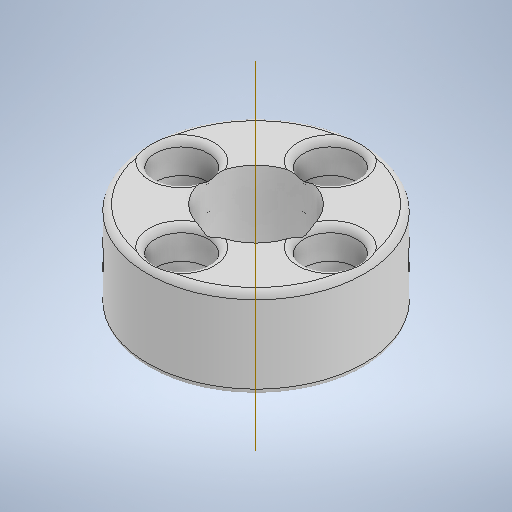
# Autodesk Inventor part: fixation_harbre_moteur_v2
Saved by Autodesk Inventor 2025.1 (Build 291241000, 241)
## iProperties
Created: 2025-05-14
Part Number: fixation_harbre_moteur_v2
Material: Générique
Document SubType Name: Modeling
Designer: chapuzet
Density: 1 g/cm^3
Appearance: Par défaut
Author: chapuzet
Autodesk Inventor part; units mm, degrees
ref_plane "XZ Plane" through (0, 0, 0) normal (0, 1, 0) x (-1, 0, 0)
sketch "Esquisse1" plane through (0, 0, 0) normal (0, 1, 0) x (-1, 0, 0)
  circle A0 centre (0, 0) radius 17.5
  circle A1 centre (0, 0) radius 12
  circle A2 centre (0, -12) radius 2
  circle A3 centre (12, 0) radius 2
  circle A4 centre (0, 12) radius 2
  circle A5 centre (-12, 0) radius 2
  dimension "d1" = 24
  dimension "d0" = 35
  dimension "d2" = 4
  dimension "d11" = 360
  constraints: 5 centre point, 2 coincident, 1 vertical alignment, 11 other
  measures "d0" diameter of A0
  measures "d2" diameter of A2
extrude "Extrusion1" add sketch "Esquisse1" along normal blind 14.5 contours A0 | A3 A1 A2 A5 A4
sketch "Esquisse2" plane through (0, 14.5, 0) normal (0, 1, 0) x (1, 0, 0)
  circle A0 centre (0, 12) radius 2 projected
  circle A1 centre (0, 12) radius 4.25
  circle A2 centre (-12, 0) radius 4.25
  circle A3 centre (0, -12) radius 4.25
  circle A4 centre (12, 0) radius 4.25
  point P0 (0, 0)
  dimension "d13" = 8.5
  dimension "d16" = 360
  constraints: 4 centre point, 1 coincident, 9 other
  measures "d13" diameter of A1
extrude "Extrusion2" cut sketch "Esquisse2" against normal blind 6
sketch "Esquisse3" plane through (0, 14.5, 0) normal (0, 1, 0) x (1, 0, 0)
  circle A0 centre (0, 0) radius 7.7
  dimension "d20" = 15.4
  constraints: 1 centre point, 1 coincident
  measures "d20" diameter of A0
extrude "Extrusion3" cut sketch "Esquisse3" against normal through all
fillet "Congé2" radius 1 14 edges at (17.5, 0, 0) (14, 0, 0) (2, 0, -12) (-10, 0, 0) (2, 0, 12) (17.5, 14.5, 0) (-16.25, 8.5, 0) (-16.25, 14.5, 0) (-4.25, 8.5, 12) (-4.25, 14.5, 12) (-4.25, 8.5, -12) (-4.25, 14.5, -12) (7.75, 8.5, 0) (7.75, 14.5, 0)
ref_plane "Plan de construction3" through (0, 0, 0) normal (0.7071068, 0, -0.7071068) x (0, 1, 0)
sketch "Esquisse7" plane through (0, 0, 0) normal (0.7071068, 0, -0.7071068) x (0, 1, 0)
  circle A0 centre (7.4335, 0) radius 2
  line L0 (0, 0) -> (14.5, 0)
  line L1 (14.5, 5.4447) -> (14.5, 5.4447) projected
  point P0 (14.5, -7.7)
  point P1 (14.5, 7.7)
  point P2 (7.25, 0)
  dimension "d53" = 14.5
  dimension "d54" = 7.25
  dimension "d55" = 4
  constraints: 2 end point, 1 centre point, 1 midpoint, 2 other
  measures "d53" distance of L0.start L0.end
  measures "d54" distance of L0.start point (7.25, 0)
  measures "d55" diameter of A0
extrude "Extrusion5" cut sketch "Esquisse7" along normal through all both and the other way through all
